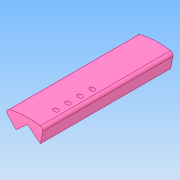
# Autodesk Inventor part: ContactMount
Saved by Autodesk Inventor 2017.3 (Build 213256000, 256)
## iProperties
Created: 2019-06-19
Part Number: ContactMount
Material: ABS Plastic
Document SubType Name: Modeling
Designer: Derek Wider
Density: 1.06 g/cm^3
Appearance: Pink
Author: Derek Wider
Autodesk Inventor part; units mm, degrees
ref_plane "YZ Plane" through (0, 0, 0) normal (1, 0, 0) x (0, 1, 0)
ref_plane "XZ Plane" through (0, 0, 0) normal (0, 1, 0) x (-1, 0, 0)
ref_plane "XY Plane" through (0, 0, 0) normal (0, 0, 1) x (1, 0, 0)
sketch "Sketch1" plane through (0, 0, 0) normal (0, 0, 1) x (1, 0, 0)
  line L0 (0, 0) -> (4.826, 4.32208)
  line L1 (4.826, 4.32208) -> (10.16, 0)
  line L2 (10.16, 0) -> (11.43, 6.221704)
  line L3 (0, 0) -> (-4.974999, 5.228953)
  arc A0 (11.43, 6.221704) -> (-4.974999, 5.228953) centre (5.08, -24.886816) ccw
  circle A1 centre (5.08, -24.886816) radius 25.4 construction
  dimension "d0" = 31.75
  dimension "d2" = 50.8
  dimension "d3" = 29.21
  dimension "d4" = 30
  dimension "d5" = 10.16
  dimension "d6" = 5.334
  constraints: 8 end point, 4 point on circle, 2 centre point, 1 coincident, 1 horizontal alignment, 1 line through centre
  measures "d0" radius of A0
  measures "d2" diameter of A1
  measures "d3" distance of A1.centre L0.end
  measures "d5" distance of L1.end L0.start
  measures "d6" horizontal distance of L1.end L0.end
extrude "Extrusion1" add sketch "Sketch1" along normal blind 54.61
fillet "Fillet1" radius 1.27 2 edges at (-4.975, 5.229, 27.305) (11.43, 6.2217, 27.305)
sketch "Sketch3" plane through (4.826, 4.32208, 0) normal (0.6671445, -0.7449283, 0) x (0.7449283, 0.6671445, 0)
  line L0 (-6.478476, 0) -> (0, 0) construction
  line L1 (0, 0) -> (0, 54.61) construction
  line L2 (-6.478476, 54.61) -> (0, 54.61) construction
  line L3 (-6.478476, 0) -> (-6.478476, 54.61) construction
  line L4 (-6.478476, 0) -> (-6.478476, 54.61)
  line L5 (0, 0) -> (0, 54.61)
  line L6 (-6.478476, 48.1584) -> (0, 48.1584)
  line L7 (0, 48.1584) -> (0, 48.6664)
  line L8 (0, 48.6664) -> (-6.478476, 48.6664)
  line L9 (-6.478476, 48.6664) -> (-6.478476, 48.1584)
  dimension "d19" = 0.508
  constraints: 8 end point, 2 parallel, 2 point on line, 1 horizontal, 1 perpendicular
  measures "d19" distance between parallel lines of L6 L8
extrude "Extrusion3" add sketch "Sketch3" along normal blind 1.524
chamfer "Chamfer1" distance 0.762 angle 45 2 edges at (2.413, 2.161, 48.6664) (2.413, 2.161, 48.1584)
pattern_linear "Rectangular Pattern3" count 5 spacing 5.08 along (0, 0, -1) of "Extrusion3", "Chamfer1"
sketch "Sketch4" plane through (10.16, 0, 0) normal (-0.6295572, -0.7769542, 0) x (0.7769542, -0.6295572, 0)
  ellipse E0 centre (-7.389761, 45.8724) end of major axis (-7.389761, 46.9519) minor radius 0.171392 construction
  ellipse E1 centre (-7.389761, 40.7924) end of major axis (-7.389761, 41.8719) minor radius 0.171392 construction
  ellipse E2 centre (-7.389761, 35.7124) end of major axis (-7.389761, 36.7919) minor radius 0.171392 construction
  ellipse E3 centre (-7.389761, 30.6324) end of major axis (-7.389761, 31.7119) minor radius 0.171392 construction
  circle A0 centre (-5.97627, 45.8724) radius 0.889
  line L0 (-6.86527, 44.3484) -> (-6.86527, 47.3964)
  point P0 (-7.893854, 0)
  point P1 (-6.86527, 45.8724)
  dimension "d31" = 1.778
  dimension "d32" = 0.889
  constraints: 1 centre point, 1 horizontal alignment, 1 midpoint, 8 other
  measures "d31" diameter of A0
  measures "d32" distance from line of L0 A0.centre
extrude "Extrusion4" cut sketch "Sketch4" against normal through all
pattern_linear "Rectangular Pattern4" count 4 spacing 5.08 along (0, 0, -1) of "Extrusion4"
sketch "Sketch6" plane through (10.16, 0, 0) normal (-0.6295572, -0.7769542, 0) x (0.7769542, -0.6295572, 0)
  line L0 (-5.360601, 48.1584) -> (-5.360601, 48.6664)
  line L1 (-5.360601, 43.0784) -> (-5.360601, 43.5864)
  line L2 (-5.360601, 37.9984) -> (-5.360601, 38.5064)
  line L3 (-5.360601, 32.9184) -> (-5.360601, 33.4264)
  line L4 (-5.360601, 27.8384) -> (-5.360601, 28.3464)
  line L5 (-5.360601, 27.8384) -> (-4.217601, 27.8384)
  line L6 (-4.217601, 27.8384) -> (-4.217601, 48.6664)
  line L7 (-4.217601, 48.6664) -> (-5.360601, 48.6664)
  line L8 (-5.360601, 48.6664) -> (-5.360601, 27.8384)
  point P0 (-7.893854, 0)
  dimension "d43" = 1.143
  constraints: 8 end point, 2 horizontal alignment, 2 parallel, 1 horizontal, 1 perpendicular
  measures "d43" distance of L4.start L5.end
extrude "Extrusion6" add sketch "Sketch6" along normal blind 5.588
chamfer "Chamfer2" distance 5.588 angle 45 1 edges at (6.4391, 3.015, 48.6664)
sketch "Sketch7" plane through (5.995059, 3.374805, 45.231095) normal (-0.7769542, 0.6295572, 0) x (0, 0, 1)
  line L0 (2.927305, -0.241965) -> (3.435305, -0.241965) construction
  line L1 (-2.152695, -0.241965) -> (-1.644695, -0.241965) construction
  line L2 (-7.232695, -0.241965) -> (-6.724695, -0.241965) construction
  line L3 (-12.312695, -0.241965) -> (-11.804695, -0.241965) construction
  line L4 (-17.392695, -0.241965) -> (-16.884695, -0.241965) construction
  line L5 (3.435305, -5.588) -> (-17.392695, -5.588) construction
  line L6 (3.435305, -0.241965) -> (2.927305, -0.241965)
  line L7 (2.927305, -0.241965) -> (2.927305, -5.588)
  line L8 (2.927305, -5.588) -> (3.435305, -5.588)
  line L9 (3.435305, -5.588) -> (3.435305, -0.241965)
  line L10 (-1.644695, -0.241965) -> (-2.152695, -0.241965)
  line L11 (-2.152695, -0.241965) -> (-2.152695, -5.550605)
  line L12 (-2.152695, -5.550605) -> (-1.644695, -5.550605)
  line L13 (-1.644695, -5.550605) -> (-1.644695, -0.241965)
  line L14 (-6.724695, -0.241965) -> (-7.232695, -0.241965)
  line L15 (-7.232695, -0.241965) -> (-7.232695, -5.588)
  line L16 (-7.232695, -5.588) -> (-6.724695, -5.588)
  line L17 (-6.724695, -5.588) -> (-6.724695, -0.241965)
  line L18 (-11.804695, -0.241965) -> (-11.804695, -6.638266)
  line L19 (-11.804695, -0.258869) -> (-12.312695, -0.258869)
  line L20 (-12.312695, -0.258869) -> (-12.312695, -5.600225)
  line L21 (-12.312695, -5.600225) -> (-11.804695, -5.600225)
  line L22 (-11.804695, -5.600225) -> (-11.804695, -0.258869)
  line L23 (-17.392695, -0.241965) -> (-17.392695, -5.588)
  line L24 (-16.884695, -0.241965) -> (-17.392695, -0.241965)
  line L25 (-17.392695, -0.241965) -> (-17.392695, -5.588)
  line L26 (-17.392695, -5.588) -> (-16.884695, -5.588)
  line L27 (-16.884695, -5.588) -> (-16.884695, -0.241965)
  point P0 (-45.231095, -6.396301)
  constraints: 40 end point, 10 parallel, 5 horizontal, 5 perpendicular, 3 point on line
extrude "Extrusion7" add sketch "Sketch7" along normal blind 2.54
chamfer "Chamfer3" distance 0.508 angle 45 9 edges at (4.1599, 1.11, 48.6664) (4.1599, 1.11, 48.1584) (4.1717, 1.1245, 43.0784) (4.1717, 1.1245, 43.5864) (4.1599, 1.11, 37.9984) (4.1599, 1.11, 38.5064) (4.1546, 1.1034, 32.9184) (4.1546, 1.1034, 33.4264) (4.1599, 1.11, 28.3464)
body "Solid1"
